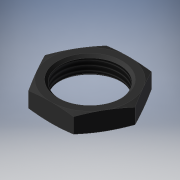
# Autodesk Inventor part: MVFKN40-NUT-NUT
Saved by Autodesk Inventor 2019 (Build 230136000, 136)
## iProperties
Created: 2023-12-16
Part Number: MVFKN40-NUT-NUT
Material: Generic
Catalog Web Link: www.cadenas.de
Description: MVPKN, MVPKE, MVPKF, MVFKN, MVFKF,MVSKS_NUT-Suction Cups - StandardType, Deep Type, Sponge Type - Fixed Type Up: One  - Touch Type (K Shape)_NUT
Vendor: MISUMI
Document SubType Name: Modeling
Designer: psAdmin
Manufacturer: MISUMI
Mass: 0.459772 g
Surface Area: 5.98784 cm^2
Volume: 0.459772 cm^3
Density: 1 g/cm^3
Appearance: PSOLRGB-175-175-175
Category: PARTsolutions
Company: MISUMI
Title: MVFKN40-NUT-NUT
Author: Cadenas PARTsolutions
Comments: Suction Cups - StandardType, Deep Type, Sponge Type - Fixed Type Up: One  - Touch Type (K Shape)_NUT
PSOL_IDENT_0: {$CADENAS_DATA/23d-libs/misumi/metric/35_tubes_nozzles/mvpkn/mvpkn_nut.prj},212 {VTYP=3D},{NB=MVFKN4
PSOL_IDENT_1: 0-NUT-NUT},{LINA=MVFKN40-NUT-NUT},{NN=MVPKN, MVPKE, MVPKF, MVFKN, MVFKF,MVSKS_NUT},{DATE=04.06.2021
PSOL_IDENT_2: 06:55:05},{GEOMDATE=06.11.2008 08:16:00},{VERSION=},{LINEID=120},{WBVAR=MATP},{WBNUMERIC=}  {NB=MVFK
PSOL_IDENT_3: N40-NUT-NUT},{LINA=MVFKN40-NUT-NUT},{KT=DUMMY},{PN=MVFKN40-NUT},{MATM=Brass},{TYPE=MVFKN},{ST=Electr
PSOL_IDENT_4: oless Nickel Plating},{AC=Suction Cup},{SHAPE=Deep},{MATP=N},{MATPALG='N', 'Nitrile Rubber','F','Flu
PSOL_IDENT_5: oro Rubber'},{NL1=40 - 17.5},{NO=40},{NO1=40},{D=6},{DD=40},{L1=17.5},{B=45.0},{L2=23.0},{L3=18.0},{
PSOL_IDENT_6: H1=17},{T=4},{M=M14x1.0},{M1=14},{M2=1.00},{L4=11.7},{MASS=47.0},{TIFF=2},{MVPNT=1},{MVPFT=1},{K1=0}
PSOL_IDENT_7: ,{K2=0},{K3=0.0},{MVPKN=1},{PLANE=17.500}
NB: MVFKN40-NUT-NUT
NN: MVPKN, MVPKE, MVPKF, MVFKN, MVFKF,MVSKS_NUT
NT: Suction Cups - StandardType, Deep Type, Sponge Type - Fixed Type Up: One  - Touch Type (K Shape)_NUT
NBSYN: $PN.-NUT
LINA: MVFKN40-NUT-NUT
CATALOG: Misumi
MATM: Brass
ST: Electroless Nickel Plating
AC: Suction Cup
SHAPE: Deep
MATP: Nitrile Rubber
NL1: 40 - 17.5
NO: 40
NO1: 40
D: 6
DD: 40
L1: 17.5
B: 45
L2: 23
L3: 18
H1: 17
T: 4
M: M14x1.0
M1: 14
M2: 1
L4: 11.7
MASS: 47
K1: 0
K2: 0
K3: 0
PLANE: 17.5
SUPPLIER: MISUMI
ARTICLENO: MVFKN40-NUT-NUT
BOMINFO: MVFKN40-NUT-NUT
CREATOR: CADENAS GmbH
Autodesk Inventor part; units mm, degrees
sketch "Sketch_1" plane through (0, 0, 0) normal (0, 0, 1) x (1, 0, 0)
  line L0 (0, 30) -> (0, 34)
  line L1 (0, 34) -> (8.5, 34)
  line L2 (8.5, 34) -> (10.2, 33.5445)
  line L3 (10.2, 33.5445) -> (10.2, 30.4555)
  line L4 (10.2, 30.4555) -> (8.5, 30)
  line L5 (8.5, 30) -> (0, 30)
  line L6 (0, 30) -> (0, 34)
  constraints: 14 end point
revolve "Revolution1" add sketch "Sketch_1" angle 360 about axis through (0, 30, 0) along (0, -1, 0)
sketch "Sketch_2" plane through (0, 0, 0) normal (0, 0, 1) x (1, 0, 0)
  line L0 (0, 30) -> (0, 34)
  line L1 (0, 34) -> (7, 34)
  line L2 (7, 34) -> (6.4585, 33.4585)
  line L3 (6.4585, 33.4585) -> (6.4585, 30.5415)
  line L4 (6.4585, 30.5415) -> (7, 30)
  line L5 (7, 30) -> (0, 30)
  line L6 (0, 30) -> (0, 34)
  constraints: 14 end point
revolve "Revolution2" cut sketch "Sketch_2" angle 360 about axis through (0, 30, 0) along (0, -1, 0)
thread "Thread1" size "M14x1" class "6H" standard "ISO Metric profile" full length
sketch "Sketch_3" plane through (0, 30, 0) normal (0, 1, 0) x (1, 0, 0)
  line L0 (-45, 45) -> (-45, -45)
  line L1 (-45, -45) -> (45, -45)
  line L2 (45, -45) -> (45, 45)
  line L3 (45, 45) -> (-45, 45)
  line L4 (-9.815, 0) -> (-4.9075, -8.5)
  line L5 (-4.9075, -8.5) -> (4.9075, -8.5)
  line L6 (4.9075, -8.5) -> (9.815, 0)
  line L7 (9.815, 0) -> (4.9075, 8.5)
  line L8 (4.9075, 8.5) -> (-4.9075, 8.5)
  line L9 (-4.9075, 8.5) -> (-9.815, 0)
  constraints: 20 end point
extrude "Extrusion1" cut sketch "Sketch_3" along normal blind 4
ref_plane "NUT_TO_BODY_XY" through (0, 30, 0) normal (0, 1, 0) x (1, 0, 0)
ref_plane "NUT_TO_BODY_YZ" through (0, 30, 0) normal (1, 0, 0) x (0, 0, -1)
ref_plane "NUT_TO_BODY_ZX" through (0, 30, 0) normal (0, 0, -1) x (0, 1, 0)
body "Solid1"
